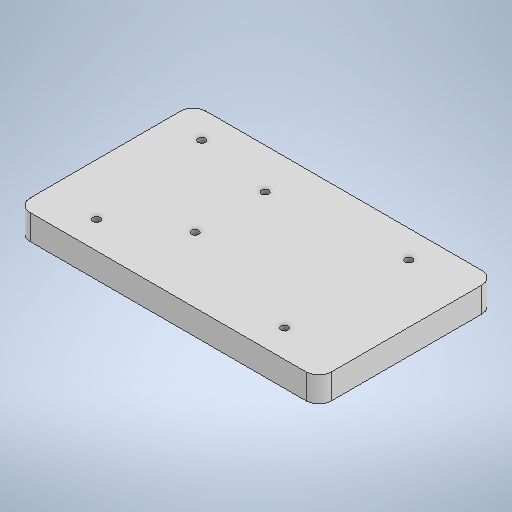
# Autodesk Inventor part: BASE ARDUINO
Saved by Autodesk Inventor 2025 (Build 290162000, 162)
## iProperties
Created: 2024-09-28
Part Number: BASE ARDUINO
Material: Genérico
Document SubType Name: Modeling
Designer: phmca
Density: 1 g/cm^3
Appearance: Padrão
Author: phmca
Autodesk Inventor part; units mm, degrees
ref_plane "YZ Plane" through (0, 0, 0) normal (1, 0, 0) x (0, 1, 0)
ref_plane "XZ Plane" through (0, 0, 0) normal (0, 1, 0) x (-1, 0, 0)
ref_plane "XY Plane" through (0, 0, 0) normal (0, 0, 1) x (1, 0, 0)
sketch "Esboço1" plane through (0, 0, 0) normal (0, 1, 0) x (-1, 0, 0)
  line L0 (-50.8, -26.605) -> (50.8, -26.605)
  line L1 (50.8, -26.605) -> (50.8, 26.605)
  line L2 (50.8, 26.605) -> (-50.8, 26.605)
  line L3 (-50.8, 26.605) -> (-50.8, -26.605)
  line L4 (-50.8, -26.605) -> (50.8, 26.605) construction
  line L5 (50.8, -26.605) -> (-50.8, 26.605) construction
  circle A0 centre (-36.83, -24.065) radius 1.45
  circle A1 centre (15.24, -18.855) radius 1.45
  circle A2 centre (45.72, -24.065) radius 1.45
  circle A3 centre (39.37, 24.195) radius 1.45
  circle A4 centre (15.24, 8.995) radius 1.45
  circle A5 centre (-35.56, 24.195) radius 1.45
  line L6 (-36.83, -24.065) -> (45.72, -24.065) construction
  line L7 (15.24, 8.995) -> (15.24, -18.855) construction
  line L8 (-35.56, 24.195) -> (39.37, 24.195)
  line L9 (-60, -35) -> (60, -35)
  line L10 (60, -35) -> (60, 35)
  line L11 (60, 35) -> (-60, 35)
  line L12 (-60, 35) -> (-60, -35)
  line L13 (-60, -35) -> (60, 35) construction
  line L14 (60, -35) -> (-60, 35) construction
  point P0 (0, 0)
  dimension "d0" = 101.6
  dimension "d1" = 53.21
  dimension "d2" = 2.9
  dimension "d3" = 2.9
  dimension "d4" = 2.9
  dimension "d5" = 2.9
  dimension "d6" = 2.9
  dimension "d7" = 2.9
  dimension "d8" = 82.55
  dimension "d9" = 66.04
  dimension "d10" = 74.93
  dimension "d11" = 48.26
  dimension "d12" = 27.85
  dimension "d13" = 7.75
  dimension "d14" = 2.54
  dimension "d15" = 13.97
  dimension "d16" = 96.52
  dimension "d17" = 15.24
  dimension "d18" = 90.17
  dimension "d19" = 120
  dimension "d20" = 70
  constraints: 30 end point, 6 centre point, 4 horizontal, 4 midpoint, 4 parallel, 2 perpendicular, 1 vertical
  measures "d0" distance of L1.end L2.end
  measures "d1" distance of L2.end L0.start
  measures "d2" diameter of A0
  measures "d3" diameter of A1
  measures "d4" diameter of A2
  measures "d5" diameter of A3
  measures "d6" diameter of A4
  measures "d7" diameter of A5
  measures "d8" distance of L6.start L6.end
  measures "d9" distance from line of L3 L7.end
  measures "d10" distance of L8.end L8.start
  measures "d11" vertical distance of L8.start L6.start
  measures "d12" distance of L7.start L7.end
  measures "d13" distance from line of L0 L7.end
  measures "d14" distance between parallel lines of L0 L6
  measures "d15" distance from line of L3 L6.start
  measures "d16" distance from line of L3 L6.end
  measures "d17" distance from line of L3 L8.start
  measures "d18" distance from line of L3 L8.end
  measures "d19" distance of L11.end L10.end
  measures "d20" distance of L10.end L9.end
extrude "Extrusão1" add sketch "Esboço1" along normal blind 10 contours L3 L2 L1 L0 | A0 | A1 | A2 | A3 | A5 | A4 | L12 L11 L10 L9
sketch "Esboço2" plane through (0, 10, 0) normal (0, 1, 0) x (1, 0, 0)
  circle A0 centre (36.83, 24.065) radius 1.45 projected
  circle A1 centre (-15.24, 18.855) radius 1.45 projected
  circle A2 centre (-45.72, 24.065) radius 1.45 projected
  circle A3 centre (-15.24, -8.995) radius 1.45 projected
  circle A4 centre (-39.37, -24.195) radius 1.45 projected
  circle A5 centre (35.56, -24.195) radius 1.45 projected
  point P0 (0, 0)
extrude "Extrusão2" cut sketch "Esboço2" against normal blind 8.5
fillet "Arredondamento1" radius 5 4 edges at (-60, 5, -35) (-60, 5, 35) (60, 5, -35) (60, 5, 35)
